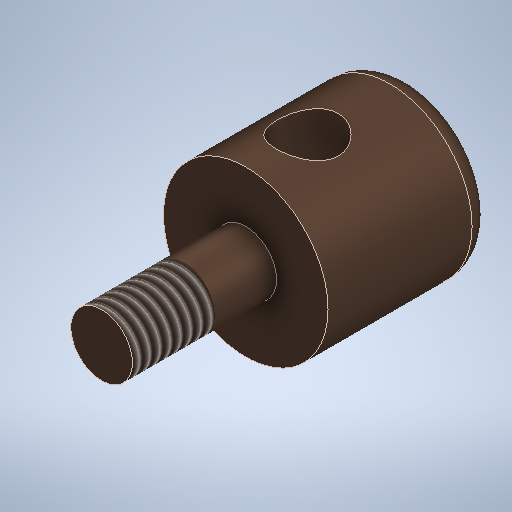
# Autodesk Inventor part: 33 - Eccentric Swivel Screw
Saved by Autodesk Inventor 2025.2 (Build 292293000, 293)
## iProperties
Created: 2025-07-30
Part Number: 33 - Eccentric Swivel Screw
Material: Bronze, Soft Tin
Document SubType Name: Modeling
Designer: bless
Density: 8.874 g/cm^3
Appearance: Bronze - Satin
Author: bless
Autodesk Inventor part; units mm, degrees
ref_plane "YZ Plane" through (0, 0, 0) normal (1, 0, 0) x (0, 1, 0)
ref_plane "XY Plane" through (0, 0, 0) normal (0, 0, 1) x (1, 0, 0)
sketch "Sketch1" plane through (0, 0, 0) normal (0, 0, 1) x (1, 0, 0)
  circle A0 centre (0, 0) radius 4
  dimension "d0" = 8
  constraints: 1 centre point, 1 coincident
  measures "d0" diameter of A0
extrude "Extrusion1" add sketch "Sketch1" against normal blind 8
sketch "Sketch2" plane through (0, 0, 0) normal (0, 0, 1) x (1, 0, 0)
  circle A0 centre (0, 0) radius 4 projected
  circle A1 centre (0, 0) radius 1.5
  dimension "d3" = 3
  constraints: 1 centre point, 1 coincident
  measures "d3" diameter of A1
extrude "Extrusion2" add sketch "Sketch2" along normal blind 7 contours A1
thread "Thread1" size "M3x0.5" class "6g" standard "ANSI Metric M Profile" length 4
fillet "Fillet1" radius 1 1 edges at (-4, 0, -8)
ref_plane "Work Plane1" through (0, 4, 0) normal (0, 1, 0) x (-1, 0, 0)
sketch "Sketch3" plane through (0, 4, 0) normal (0, 1, 0) x (-1, 0, 0)
  line L0 (4, 0) -> (-4, 0) projected
  line L1 (-4, -7) -> (4, -7) projected
  arc A0 (0, 0) -> (0, 0) centre (3, -7) ccw projected
  line L2 (3, -8) -> (-3, -8) projected
  line L3 (4, 0) -> (4, -7) projected
  line L4 (-4, 0) -> (-4, -7) projected
  point P0 (0, -3)
  point P1 (0, -8)
  dimension "d10" = 5
  dimension "d11" = 4
  constraints: 1 midpoint
  measures "d10" distance of point (0, -3) point (0, -8)
  measures "d11" distance from line of L3 point (0, -3)
hole "Hole1" at (0, 4, -3) direction (0, -1, 0) diameter 3 end through all
body "Solid1"
